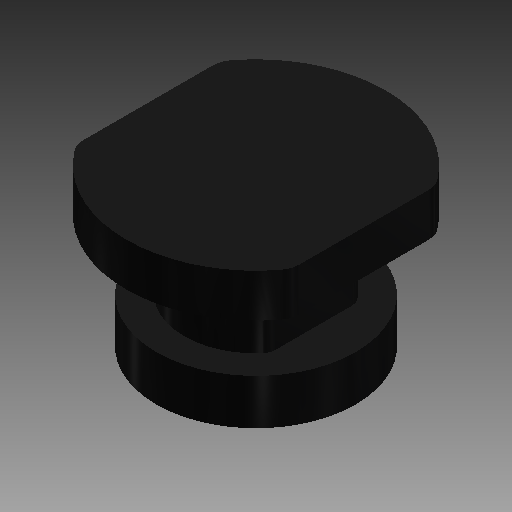
# Autodesk Inventor part: 318-06
Saved by Autodesk Inventor 2019 (Build 230136000, 136)
## iProperties
Company: Autodesk Inc.
Created: 2007-10-25
Part Number: 318-06
Document SubType Name: Modeling
Designer: Autodesk Inc.
Density: 7.85 g/cm^3
Mass: 11.888 g
Surface Area: 10.7782 cm^2
Volume: 1.51439 cm^3
Material: Steel
Description: CONNECTOR PIN
Appearance: Glossy - Black
Component Category: Fasteners
Author: Inventor
Autodesk Inventor part; units mm, degrees
ref_plane "YZ Plane" through (0, 0, 0) normal (1, 0, 0) x (0, 1, 0)
ref_plane "XZ Plane" through (0, 0, 0) normal (0, 1, 0) x (-1, 0, 0)
ref_plane "XY Plane" through (0, 0, 0) normal (0, 0, 1) x (1, 0, 0)
sketch "Sketch1" plane through (0, 0, 0) normal (0, 0, 1) x (1, 0, 0)
  line L0 (0, 0) -> (0, -10.95)
  line L1 (0, -10.95) -> (6.925, -10.95)
  line L2 (6.925, -10.95) -> (6.925, -7.8)
  line L3 (6.925, -7.8) -> (5, -7.8)
  line L4 (5, -7.8) -> (5, -3)
  line L5 (5, -3) -> (9, -3)
  line L6 (9, -3) -> (9, 0)
  line L7 (9, 0) -> (0, 0)
  dimension "d0" = 6.925
  dimension "d1" = 5
  dimension "d2" = 9
  dimension "d3" = 3.15
  dimension "d4" = 4.8
  dimension "d5" = 3
  constraints: 16 end point, 6 parallel, 1 perpendicular, 1 vertical
  measures "d0" distance of L0.end L1.end
  measures "d1" distance between parallel lines of L0 L4
  measures "d2" distance between parallel lines of L0 L6
  measures "d3" distance of L1.end L2.end
  measures "d4" distance of L3.end L4.end
  measures "d5" distance of L5.end L6.end
revolve "Revolution1" add sketch "Sketch1" angle 360 about axis through (0, 0, 0) along (0, -1, 0)
sketch "Sketch2" plane through (0, 0, 0) normal (0, 1, 0) x (1, 0, 0)
  circle A0 centre (0, 0) radius 9 projected
  line L0 (0, 12.6) -> (0, -12.6) projected
  line L1 (7.5, 4.9749) -> (7.5, -4.9749)
  line L2 (-7.5, 4.9749) -> (-7.5, -4.9749)
  dimension "d7" = 15
  dimension "d8" = 7.5
  constraints: 4 end point, 4 point on circle, 2 parallel
  measures "d7" distance between parallel lines of L2 L1
  measures "d8" distance between parallel lines of L0 L2
extrude "Extrusion1" cut sketch "Sketch2" against normal up to surface (3 mm away) contours A0 L1 | L2 A0
sketch "Sketch3" plane through (0, -3, 0) normal (0, -1, 0) x (1, 0, 0)
  arc A0 (-7.5, -4.9749) -> (7.5, -4.9749) centre (0, 0) ccw projected
  line L0 (7.5, -4.9749) -> (7.5, 4.9749) projected
  circle A1 centre (0, 0) radius 5 projected
  line L1 (-4, -3) -> (-4, 3)
  line L2 (4, -3) -> (4, 3)
  dimension "d11" = 8
  dimension "d12" = 4
  constraints: 4 end point, 4 point on circle, 2 parallel
  measures "d11" distance between parallel lines of L2 L1
  measures "d12" distance from line of A0.centre L2
extrude "Extrusion2" cut sketch "Sketch3" along normal up to surface (4.8 mm away) contours A1 L2 | L1 A1
fillet "Fillet1" radius 1 4 edges at (4, -5.4, 3) (4, -5.4, -3) (-4, -5.4, 3) (-4, -5.4, -3)
fillet "Fillet2" radius 1.5 4 edges at (7.5, -1.5, 4.9749) (7.5, -1.5, -4.9749) (-7.5, -1.5, 4.9749) (-7.5, -1.5, -4.9749)
equation "\"d8\" = 0.5 * d7"
equation "\"d12\" = 0.5 * d11"
body "Solid1"
